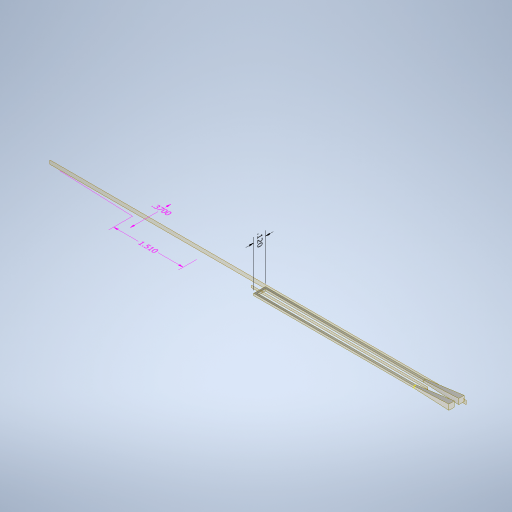
# Autodesk Inventor part: basic strain gauge 0p02
Saved by Autodesk Inventor 2024.2 (Build 282272000, 272)
## iProperties
Created: 2024-07-17
Part Number: basic strain gauge 0p02
Material: Silver
Document SubType Name: Modeling
Designer: Makerspace
Density: 10.49 g/cm^3
Appearance: Silver
Author: Makerspace
Autodesk Inventor part; units mm, degrees
ref_plane "XZ Plane" through (0, 0, 0) normal (0, 1, 0) x (-1, 0, 0)
sketch "Sketch1" plane through (0, 0, 0) normal (0, 1, 0) x (-1, 0, 0)
  line L0 (0, 0) -> (41.275, 0)
  line L1 (41.275, -2.54) -> (0, -2.54)
  line L2 (41.275, -2.54) -> (41.275, 0)
  dimension "d69" = 41.275
  dimension "d70" = 41.275
  dimension "d89" = 2.54
  dimension "d90" = 0
  dimension "d91" = 0
  dimension "d92" = 0
  constraints: 6 end point, 1 horizontal, 1 vertical
  measures "d69" distance of L1.start L1.end
  measures "d70" distance of L0.start L0.end
  measures "d89" distance of L1.start L0.end
  measures "d90" distance of point (0, 0) L0.start
  measures "d91" horizontal distance of point (0, 0) L1.end
  measures "d92" distance of point (0, 0) L0.start
sketch "Sketch2" plane through (0, 0, 0) normal (1, 0, 0) x (0, 1, 0)
  line L0 (-0.254, 0.254) -> (0.254, 0.254)
  line L1 (0.254, 0.254) -> (0.254, -0.254)
  line L2 (0.254, -0.254) -> (-0.254, -0.254)
  line L3 (-0.254, -0.254) -> (-0.254, 0.254)
  dimension "d98" = 0.508
  dimension "d99" = 0.508
  constraints: 8 end point, 2 parallel, 1 horizontal, 1 perpendicular
  measures "d98" distance of L0.end L1.end
  measures "d99" distance of L1.end L2.end
sweep "Sweep1" add profiles "Sketch2" path "Sketch1" path curves L0 L2 L1
ref_plane "Work Plane1" through (9.525, 0, 0) normal (1, 0, 0) x (0, 1, 0)
ref_plane "Work Plane2" through (0, 0, -6.35) normal (0, 0, 1) x (1, 0, 0)
ref_plane "Work Plane4" through (0, 0, -2.9845) normal (0, 0, 1) x (1, 0, 0)
sketch "Sketch15" plane through (9.525, 0, 0) normal (1, 0, 0) x (0, 1, 0)
  line L0 (-0.254, -0.254) -> (-0.254, -2.286) projected
  line L1 (1.143, 0.6985) -> (-0.254, 0.6985)
  line L2 (-0.254, 0.6985) -> (-0.254, -0.6985)
  line L3 (-0.254, -0.6985) -> (1.143, -0.6985)
  line L4 (1.143, -0.6985) -> (1.143, 0.6985)
  line L5 (0.254, -2.286) -> (-0.254, -2.286) projected
  line L6 (-0.254, -2.286) -> (-0.254, -2.794) projected
  point P0 (0, 0)
  point P1 (1.143, 0)
  point P2 (0, -2.286)
  point P3 (0.635, -2.286)
  dimension "d100" = 1.397
  dimension "d102" = 1.397
  dimension "d104" = 0
  constraints: 8 end point, 2 midpoint, 2 parallel, 1 horizontal, 1 perpendicular, 1 point on line
  measures "d100" distance of L2.end L3.end
  measures "d102" distance of L3.end L1.start
  measures "d104" vertical distance of point (0, 0) point (1.143, 0)
sketch "Sketch16" plane through (0, -0.254, -0.254) normal (1, 0, 0) x (0, 0, -1)
  line L0 (0, 0) -> (0, 0.508) projected
  line L1 (0, 0.508) -> (-0.508, 0.508) projected
  line L2 (-0.508, 0.508) -> (-0.508, 0) projected
  line L3 (-0.508, 0) -> (0, 0) projected
  point P0 (-0.254, 0.254)
loft "Loft3" add profiles "Sketch15" section 2 edges at (0, 0, -0.254) (0, 0.254, 0) (0, 0, 0.254) (0, -0.254, 0)
ref_plane "Work Plane5" through (-41.529, 0.254, -1.27) normal (0, 0, 1) x (1, 0, 0)
mirror "Mirror3" about plane through (-41.529, 0.254, -1.27) normal (0, 0, 1) of "Loft3"
body "Solid1"
